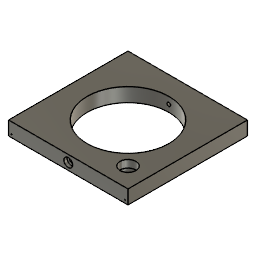
BATI (Autodesk Fusion 360 design; units mm, degrees)
Autodesk Fusion 360 part; units mm, degrees
sketch "Esquisse1" plane through (0, 0, 0) normal (0, 0, 1) x (1, 0, 0)
  line L0 (-150, 150) -> (150, 150)
  line L1 (150, 150) -> (150, -150)
  line L2 (150, -150) -> (-150, -150)
  line L3 (-150, -150) -> (-150, 150)
  constraint horizontal L0
  constraint vertical L1
  constraint horizontal L2
  constraint vertical L3
extrude "Extrusion1" add sketch "Esquisse1" along normal blind 35
sketch "Esquisse2" plane through (0, -150, 0) normal (0, -1, 0) x (1, 0, 0)
  line L0 (-150, 0) -> (150, 0)
  line L1 (150, 0) -> (150, 35)
  line L2 (150, 35) -> (-150, 35)
  line L3 (-150, 35) -> (-150, 0)
  line L4 (-150, 0) -> (-300, -210)
  line L5 (-300, -210) -> (-350, -210)
  line L6 (-350, -210) -> (-150, 35)
  constraint coincident L0.start L3.end
  constraint perpendicular L3 L5
  constraint coincident L2.end L3.start
sketch "Esquisse3" plane through (0, 0, 35) normal (0, 0, 1) x (-1, 0, 0)
  line L0 (150, 150) -> (-150, 150)
  line L1 (-150, 150) -> (-150, -150)
  line L2 (-150, -150) -> (150, -150)
  line L3 (150, -150) -> (150, 150)
  circle A0 through (11, 150, -17.5) (-5.5, 150, -7.9737) (-5.5, 150, -27.0263)
  line L4 (150, 150, -35) -> (-150, 150, -35)
  line L5 (-150, 150, -35) -> (-150, 150, 0)
  line L6 (-150, 150) -> (150, 150)
  line L7 (150, 150, 0) -> (150, 150, -35)
  dimension "d3" = 22
extrude "Extrusion2" cut sketch "Esquisse3" against normal blind 8 contours A0 in plane through (0, -150, 35) normal (0, -1, 0)
sketch "Esquisse4" plane through (0, 0, 35) normal (0, 0, 1) x (-1, 0, 0)
  line L0 (150, 150) -> (-150, 150)
  line L1 (-150, 150) -> (-150, -150)
  line L2 (-150, -150) -> (150, -150)
  line L3 (150, -150) -> (150, 150)
  circle A0 centre (0, 0) radius 102.5
  dimension "d6" = 205
  constraint coincident A0.centre origin
  measures "d6" diameter of A0
extrude "Extrusion3" cut sketch "Esquisse4" against normal blind 35 contours A0
hole "Perçage1" at (0, -142, 17.5) direction (0, 1, 0) diameter 9 depth 55 tip angle 180
sketch "Esquisse5" plane through (0, 150, 0) normal (0, 1, 0) x (-1, 0, 0)
  line L0 (-150, 0) -> (150, 0)
  line L1 (150, 0) -> (150, 35)
  line L2 (150, 35) -> (-150, 35)
  line L3 (-150, 35) -> (-150, 0)
  line L4 (-150, 0) -> (-300, -210)
  line L5 (-300, -210) -> (-350, -210)
  line L6 (-350, -210) -> (-150, 35)
  constraint coincident L0.start L3.end
  constraint horizontal L5
  constraint coincident L2.end L3.start
sketch "Esquisse6" plane through (0, 150, 0) normal (0, 1, 0) x (-1, 0, 0)
  circle A0 centre (0, 17.5) radius 11
  dimension "d12" = 22
  measures "d12" diameter of A0
extrude "Extrusion4" cut sketch "Esquisse6" against normal blind 8
hole "Perçage2" at (0, 142, 17.5) direction (0, -1, 0) diameter 9 depth 55 tip angle 118
sketch "Esquisse7" plane through (0, 0, 35) normal (0, 0, 1) x (-1, 0, 0)
  circle A0 centre (0, 0) radius 102.5
  line L0 (150, 150) -> (-150, 150)
  line L1 (-150, 150) -> (-150, -150)
  line L2 (-150, -150) -> (150, -150)
  line L3 (150, -150) -> (150, 150)
  circle A1 centre (-100, 100) radius 20
form "Forme1" [no effect]
extrude "Extrusion5" cut sketch "Esquisse7" against normal blind 18.75 contours A1
sphere "SpherePrimitive1" cut diameter 40 placed x (-1, 0, 0) y (0, -1, 0) z (0, 0, 1) at (100, -100, 16.25)
extrude "Extrusion6" add sketch "Esquisse2" against normal blind 50 contours L3 L4 L5 L6
extrude "Extrusion7" add sketch "Esquisse5" against normal blind 50 contours L3 L4 L5 L6
sketch "Esquisse9" plane through (0, 150, 0) normal (0, 1, 0) x (-1, 0, 0)
  circle A0 centre (0, 17.5) radius 11
  line L0 (-150, 0) -> (150, 0)
  line L1 (150, 0) -> (150, 35)
  line L2 (150, 35) -> (-150, 35)
  line L3 (-150, 35) -> (-350, -210)
  line L4 (-350, -210) -> (-300, -210)
  line L5 (-300, -210) -> (-150, 0)
  line L6 (150, 0) -> (300, -210)
  line L7 (300, -210) -> (350, -210)
  line L8 (350, -210) -> (150, 35)
  constraint coincident L0.end L1.start
  constraint perpendicular L1 L7
  constraint coincident L1.end L2.start
extrude "Extrusion8" add sketch "Esquisse9" against normal blind 50 contours L1 L6 L7 L8
sketch "Esquisse10" plane through (0, 0, 35) normal (0, 0, 1) x (-1, 0, 0)
  circle A0 centre (-100, 100) radius 20
  circle A1 centre (0, 0) radius 102.5
  line L0 (150, 150) -> (-150, 150)
  line L1 (-150, 150) -> (-150, -100)
  line L2 (-150, -100) -> (-150, -150)
  line L3 (-150, -150) -> (150, -150)
  line L4 (150, -150) -> (150, -100)
  line L5 (150, -100) -> (150, 100)
  line L6 (150, 100) -> (150, 150)
  line L7 (-150, -100, 0) -> (-150, -100, -35)
  line L8 (-150, -100, -35) -> (-300, -100, -245)
  line L9 (-300, -100, -245) -> (-350, -100, -245)
  line L10 (-350, -100, -245) -> (-150, -100, 0)
  point P0 (-150, -100)
  point P1 (-300, -100)
  point P2 (-350, -100)
  constraint coincident P0 L1.end
extrude "Extrusion9" add sketch "Esquisse10" along normal blind 250 contours L7 L8 L9 L10 in plane through (0, 100, 35) normal (0, -1, 0)
extrude "Extrusion10" cut 1 faces at (-266.6667, 100, -140) along direction (0, -1, 0) blind 250
extrude "Extrusion11" add 1 faces at (-266.6667, 100, -140) along direction (0, -1, 0) blind 250
extrude "Extrusion12" add 1 faces at (316.6667, 50, -210) along direction (0, 0, -1) blind 100
extrude "Extrusion13" add 1 faces at (-333.3333, -50, -210) along direction (0, 0, -1) blind 100
sketch "Esquisse11" plane through (0, -150, 0) normal (0, -1, 0) x (1, 0, 0)
  line L0 (-150, 0) -> (150, 0)
  line L1 (150, 0) -> (300, -210)
  line L2 (300, -210) -> (300, -310)
  line L3 (300, -310) -> (350, -310)
  line L4 (350, -310) -> (350, -210)
  line L5 (350, -210) -> (150, 35)
  line L6 (150, 35) -> (-150, 35)
  line L7 (-150, 35) -> (-350, -210)
  line L8 (-350, -210) -> (-350, -310)
  line L9 (-350, -310) -> (-300, -310)
  line L10 (-300, -310) -> (-300, -210)
  line L11 (-300, -210) -> (-150, 0)
  circle A0 centre (0, 17.5) radius 11
  line L12 (-150, 0) -> (-300, -210)
  line L13 (-300, -310) -> (-350, -310)
  line L14 (-350, -210) -> (-150, 35)
  line L15 (-150, 35) -> (-400, 35)
  line L16 (-400, 35) -> (-400, -350)
  line L17 (-400, -350) -> (-150, -350)
  line L18 (-150, -350) -> (-150, 35)
  constraint coincident L0.start L11.end
  constraint coincident L10.end L11.start
  constraint coincident L9.end L10.start
  constraint coincident L8.end L9.start
  constraint coincident L7.end L8.start
  constraint coincident L6.end L7.start
  constraint horizontal L15
  constraint vertical L16
  constraint horizontal L17
  constraint vertical L18
extrude "Extrusion14" cut sketch "Esquisse11" against normal blind 300 contours L7 L8 L9 L10 L11 L12 L13 L14 L18
sketch "Esquisse12" plane through (0, 0, 0) normal (0, 1, 0) x (1, 0, 0)
  line L0 (150, -35, -150) -> (150, 0, -150)
  line L1 (150, 0, -150) -> (300, 210, -150)
  line L2 (300, 210, -150) -> (300, 310, -150)
  line L3 (150, -35, -150) -> (350, 210, -150)
  line L4 (350, 210, -150) -> (350, 310, -150)
  line L5 (350, 310, -150) -> (300, 310, -150)
  point P0 (150, -35)
  point P1 (150, 0)
  point P2 (300, 210)
  point P3 (300, 310)
  point P4 (350, 210)
  point P5 (350, 310)
extrude "Extrusion15" cut sketch "Esquisse12" along normal blind 300 contours L0 L1 L2 L3 L4 L5 in plane through (0, -150, 0) normal (0, 1, 0)
sketch "Esquisse13" plane through (0, -150, 0) normal (0, -1, 0) x (1, 0, 0)
  line L0 (150, 0) -> (150, 35)
  line L1 (150, 35) -> (-150, 35)
  line L2 (-150, 35) -> (-150, 0)
  line L3 (-150, 0) -> (150, 0)
  circle A0 centre (0, 17.5) radius 11
  line L4 (150, 0) -> (135, 0)
  line L5 (135, 0) -> (135, 15)
  line L6 (135, 15) -> (150, 15)
  line L7 (150, 15) -> (150, 0)
  constraint horizontal L4
  constraint vertical L5
  constraint horizontal L6
  constraint vertical L7
  constraint coincident L0.start L3.end
extrude "Extrusion16" cut sketch "Esquisse13" against normal blind 15 contours L0 L3 L4 L5 L6 L7
sketch "Esquisse14" plane through (0, 0, 0) normal (0, 0, -1) x (1, 0, 0)
  line L0 (135, 135) -> (135, 150)
  line L1 (135, 150) -> (-150, 150)
  line L2 (-150, 150) -> (-150, -150)
  line L3 (-150, -150) -> (150, -150)
  line L4 (150, -150) -> (150, 135)
  line L5 (150, 135) -> (135, 135)
  circle A0 centre (100, 100) radius 11.6592
  circle A1 centre (0, 0) radius 102.5
  line L6 (-150, 150) -> (-135, 150)
  line L7 (-135, 150) -> (-135, 135)
  line L8 (-135, 135) -> (-150, 135)
  line L9 (-150, 135) -> (-150, 150)
  constraint horizontal L6
  constraint vertical L7
  constraint horizontal L8
  constraint vertical L9
  constraint coincident L1.end L2.start
extrude "Extrusion17" cut sketch "Esquisse14" against normal blind 15 contours L1 L2 L6 L7 L8 L9
sketch "Esquisse15" plane through (0, 150, 0) normal (0, 1, 0) x (-1, 0, 0)
  circle A0 centre (0, 17.5) radius 11
  line L0 (-150, 35) -> (-150, 0)
  line L1 (-150, 0) -> (150, 0)
  line L2 (150, 0) -> (150, 35)
  line L3 (150, 35) -> (-150, 35)
  line L4 (-150, 0) -> (-135, 0)
  line L5 (-135, 0) -> (-135, 15)
  line L6 (-135, 15) -> (-150, 15)
  line L7 (-150, 15) -> (-150, 0)
  constraint horizontal L4
  constraint vertical L5
  constraint horizontal L6
  constraint vertical L7
  constraint coincident L0.end L1.start
extrude "Extrusion18" cut sketch "Esquisse15" against normal blind 15 contours L0 L1 L4 L5 L6 L7
sketch "Esquisse16" plane through (0, 0, 0) normal (0, 0, -1) x (1, 0, 0)
  line L0 (135, -150) -> (135, -135)
  line L1 (135, -135) -> (150, -135)
  line L2 (150, -135) -> (150, 135)
  line L3 (150, 135) -> (135, 135)
  line L4 (135, 135) -> (135, 150)
  line L5 (135, 150) -> (-135, 150)
  line L6 (-135, 150) -> (-135, 135)
  line L7 (-135, 135) -> (-150, 135)
  line L8 (-150, 135) -> (-150, -150)
  line L9 (-150, -150) -> (135, -150)
  circle A0 centre (100, 100) radius 11.6592
  circle A1 centre (0, 0) radius 102.5
  line L10 (-150, -150) -> (-135, -150)
  line L11 (-135, -150) -> (-135, -135)
  line L12 (-135, -135) -> (-150, -135)
  line L13 (-150, -135) -> (-150, -150)
  constraint horizontal L10
  constraint vertical L11
  constraint horizontal L12
  constraint vertical L13
  constraint coincident L8.end L9.start
extrude "Extrusion19" cut sketch "Esquisse16" against normal blind 15 contours L8 L9 L10 L11 L12 L13
hole "Perçage3" at (-142.5, -142.5, 15) direction (0, 0, 1) diameter 2.529 depth 6 tip angle 118
thread "Filetage1" "ISO Metric profile 3.0 M3x0.5 M3x0.5 6H" thread offset 0 thread depth 7.4
hole "Perçage4" at (-142.5, -135, 7.5) direction (0, 1, 0) diameter 2.529 depth 6 tip angle 118
thread "Filetage2" "ISO Metric profile 3.0 M3x0.5 M3x0.5 6H" thread offset 0 thread depth 7.4
hole "Perçage5" at (-135, -142.5, 7.5) direction (1, 0, 0) diameter 2.529 depth 6 tip angle 118
thread "Filetage3" "ISO Metric profile 3.0 M3x0.5 M3x0.5 6H" thread offset 0 thread depth 7.4
hole "Perçage6" at (135, -142.5, 7.5) direction (-1, 0, 0) diameter 2.529 depth 6 tip angle 118
thread "Filetage4" "ISO Metric profile 3.0 M3x0.5 M3x0.5 6H" thread offset 0 thread depth 7.4
hole "Perçage7" at (142.5, -142.5, 15) direction (0, 0, 1) diameter 2.529 depth 6 tip angle 118
thread "Filetage5" "ISO Metric profile 3.0 M3x0.5 M3x0.5 6H" thread offset 0 thread depth 7.4
hole "Perçage8" at (142.5, -135, 7.5) direction (0, 1, 0) diameter 2.529 depth 6 tip angle 118
thread "Filetage6" "ISO Metric profile 3.0 M3x0.5 M3x0.5 6H" thread offset 0 thread depth 7.4
hole "Perçage9" at (135, 142.5, 7.5) direction (-1, 0, 0) diameter 2.529 depth 6 tip angle 118
thread "Filetage7" "ISO Metric profile 3.0 M3x0.5 M3x0.5 6H" thread offset 0 thread depth 7.4
hole "Perçage10" at (142.5, 142.5, 15) direction (0, 0, 1) diameter 2.529 depth 6 tip angle 118
thread "Filetage8" "ISO Metric profile 3.0 M3x0.5 M3x0.5 6H" thread offset 0 thread depth 7.4
hole "Perçage11" at (142.5, 135, 7.5) direction (0, -1, 0) diameter 2.529 depth 6 tip angle 118
thread "Filetage9" "ISO Metric profile 3.0 M3x0.5 M3x0.5 6H" thread offset 0 thread depth 7.4
hole "Perçage12" at (-142.5, 135, 7.5) direction (0, -1, 0) diameter 2.529 depth 6 tip angle 118
thread "Filetage10" "ISO Metric profile 3.0 M3x0.5 M3x0.5 6H" thread offset 0 thread depth 7.4
hole "Perçage13" at (-135, 142.5, 7.5) direction (1, 0, 0) diameter 2.529 depth 6 tip angle 118
thread "Filetage11" "ISO Metric profile 3.0 M3x0.5 M3x0.5 6H" thread offset 0 thread depth 7.4
hole "Perçage14" at (-142.5, 142.5, 15) direction (0, 0, 1) diameter 2.529 depth 6 tip angle 118
thread "Filetage12" "ISO Metric profile 3.0 M3x0.5 M3x0.5 6H" thread offset 0 thread depth 7.4
delete_face "DeleteFace1" 1 faces at (133, -143.4052, 8.3829)
delete_face "DeleteFace2" 1 faces at (141.2359, -142.5315, 17)
extrude "Extrusion20" add 1 faces at (137.0797, -135, 7.4685) along direction (0, -1, 0) blind 15
delete_face "DeleteFace3" 1 faces at (-143.7641, -142.5315, 17)
delete_face "DeleteFace4" 1 faces at (-133, -143.4052, 8.3829)
extrude "Extrusion21" add 1 faces at (-137.0797, -135, 7.5315) along direction (0, -1, 0) blind 15
delete_face "DeleteFace5" 1 faces at (141.2359, 142.4685, 17)
delete_face "DeleteFace6" 1 faces at (133, 141.5948, 8.3829)
extrude "Extrusion22" add 1 faces at (147.9203, 135, 7.4685) along direction (0, 1, 0) blind 15
delete_face "DeleteFace7" 1 faces at (-143.7641, 142.4685, 17)
delete_face "DeleteFace8" 1 faces at (-133, 141.5948, 8.3829)
extrude "Extrusion23" add 1 faces at (-137.0797, 135, 7.5315) along direction (0, 1, 0) blind 15
equation "d19 = ( -37.5 / 2 ) * 1 mm"
